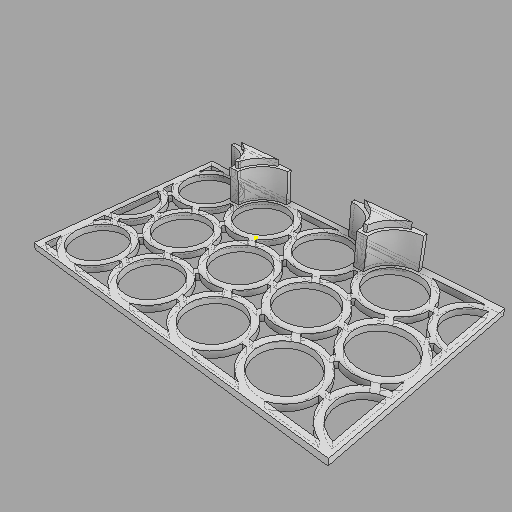
# Autodesk Inventor part: TubeHolder
Saved by Autodesk Inventor 2025 (Build 290162010, 162A)
## iProperties
Created: 2025-03-06
Part Number: TubeHolder
Material: Generic
Document SubType Name: Modeling
Designer: schanen
Density: 1 g/cm^3
Appearance: Default
Author: schanen
Autodesk Inventor part; units mm, degrees
ref_plane "YZ Plane" through (0, 0, 0) normal (1, 0, 0) x (0, 1, 0)
ref_plane "XZ Plane" through (0, 0, 0) normal (0, 1, 0) x (-1, 0, 0)
ref_plane "XY Plane" through (0, 0, 0) normal (0, 0, 1) x (1, 0, 0)
sketch "Sketch1" plane through (0, 0, 0) normal (0, 1, 0) x (-1, 0, 0)
  line L0 (-47.5, 29.5) -> (47.5, 29.5)
  line L1 (47.5, 29.5) -> (47.5, -29.5)
  line L2 (47.5, -29.5) -> (-47.5, -29.5)
  line L3 (-47.5, -29.5) -> (-47.5, 29.5)
  line L4 (-47.5, 29.5) -> (47.5, -29.5) construction
  line L5 (47.5, 29.5) -> (-47.5, -29.5) construction
  circle A0 centre (36.75, -18.1865) radius 8
  line L6 (36.75, -18.1865) -> (23.7803, 4.2776)
  circle A1 centre (26.25, 0) radius 8
  circle A2 centre (15.75, 18.1865) radius 8
  circle A3 centre (15.75, -18.1865) radius 8
  circle A4 centre (5.25, 0) radius 8
  circle A5 centre (-5.25, 18.1865) radius 8
  circle A6 centre (57.75, -18.1865) radius 8
  circle A7 centre (47.25, 0) radius 8
  circle A8 centre (36.75, 18.1865) radius 8
  circle A9 centre (-5.25, -18.1865) radius 8
  circle A10 centre (-15.75, 0) radius 8
  circle A11 centre (-26.25, 18.1865) radius 8
  circle A12 centre (78.75, -18.1865) radius 8
  circle A13 centre (68.25, 0) radius 8
  circle A14 centre (57.75, 18.1865) radius 8
  circle A15 centre (-26.25, -18.1865) radius 8
  circle A16 centre (-36.75, 0) radius 8
  circle A17 centre (-47.25, 18.1865) radius 8
  circle A18 centre (36.75, -18.1865) radius 10
  circle A19 centre (26.25, 0) radius 10
  circle A20 centre (15.75, 18.1865) radius 10
  circle A21 centre (15.75, -18.1865) radius 10
  circle A22 centre (5.25, 0) radius 10
  circle A23 centre (-5.25, 18.1865) radius 10
  circle A24 centre (57.75, -18.1865) radius 10
  circle A25 centre (47.25, 0) radius 10
  circle A26 centre (36.75, 18.1865) radius 10
  circle A27 centre (-5.25, -18.1865) radius 10
  circle A28 centre (-15.75, 0) radius 10
  circle A29 centre (-26.25, 18.1865) radius 10
  circle A30 centre (78.75, -18.1865) radius 10
  circle A31 centre (68.25, 0) radius 10
  circle A32 centre (57.75, 18.1865) radius 10
  circle A33 centre (-26.25, -18.1865) radius 10
  circle A34 centre (-36.75, 0) radius 10
  circle A35 centre (-47.25, 18.1865) radius 10
  line L7 (-45.5, 27.5) -> (45.5, 27.5)
  line L8 (45.5, 27.5) -> (45.5, -27.5)
  line L9 (45.5, -27.5) -> (-45.5, -27.5)
  line L10 (-45.5, -27.5) -> (-45.5, 27.5)
  line L11 (-45.5, 27.5) -> (45.5, -27.5) construction
  line L12 (45.5, 27.5) -> (-45.5, -27.5) construction
  circle A36 centre (99.75, -18.1865) radius 8
  circle A37 centre (89.25, 0) radius 8
  circle A38 centre (78.75, 18.1865) radius 8
  circle A39 centre (-47.25, -18.1865) radius 8
  circle A40 centre (-57.75, 0) radius 8
  circle A41 centre (-68.25, 18.1865) radius 8
  circle A42 centre (99.75, -18.1865) radius 10
  circle A43 centre (89.25, 0) radius 10
  circle A44 centre (78.75, 18.1865) radius 10
  circle A45 centre (-47.25, -18.1865) radius 10
  circle A46 centre (-57.75, 0) radius 10
  circle A47 centre (-68.25, 18.1865) radius 10
  point P0 (0, 0)
  point P1 (45.5, -23.0278)
  point P2 (40.3913, -27.5)
  point P3 (40.3913, 27.5)
  point P4 (45.5, 23.0278)
  point P5 (45.5, -13.3453)
  point P6 (33.1087, -27.5)
  point P7 (19.3913, -27.5)
  point P8 (12.1087, -27.5)
  point P9 (-1.6087, -27.5)
  point P10 (-8.8913, -27.5)
  point P11 (-22.6087, -27.5)
  point P12 (-29.8913, -27.5)
  point P13 (-45.5, -4.8412)
  point P14 (-45.5, 4.8412)
  point P15 (-29.8913, 27.5)
  point P16 (-22.6087, 27.5)
  point P17 (-8.8913, 27.5)
  point P18 (-1.6087, 27.5)
  point P19 (12.1087, 27.5)
  point P20 (19.3913, 27.5)
  point P21 (33.1087, 27.5)
  point P22 (45.5, 13.3453)
  point P23 (-45.5, 25.9928)
  point P24 (-45.5, 10.3803)
  point P25 (-45.5, 8.3408)
  point P26 (-43.6087, 27.5)
  point P27 (-45.5, -8.3408)
  point P28 (-45.5, -10.3803)
  point P29 (-45.5, -25.9928)
  point P30 (-43.6087, -27.5)
  point P31 (45.5, -9.8457)
  point P32 (45.5, -7.8062)
  point P33 (45.5, 7.8062)
  point P34 (45.5, 9.8457)
  dimension "d0" = 95
  dimension "d1" = 59
  dimension "d2" = 16
  dimension "d3" = 60
  dimension "d6" = 21
  dimension "d9" = 21
  dimension "d12" = 11.3135
  dimension "d13" = 10.75
  dimension "d14" = 36.3731
  dimension "d15" = 20
  dimension "d18" = 21
  dimension "d21" = 21
  dimension "d24" = 2
  dimension "d25" = 2
  constraints: 48 centre point, 26 end point, 4 horizontal, 4 midpoint, 4 parallel, 2 perpendicular, 1 coincident, 94 other
  measures "d0" distance of L1.end L2.end
  measures "d1" distance of L0.end L1.end
  measures "d2" diameter of A0
  measures "d3" angle of L2 L6
  measures "d6" distance of L6.start A1.centre
  measures "d9" distance of L6.start A3.centre
  measures "d12" distance from line of L2 L6.start
  measures "d13" distance from line of L1 L6.start
  measures "d14" distance of A11.centre A15.centre
  measures "d15" diameter of A18
  measures "d18" distance of A18.centre A19.centre
  measures "d21" distance of A18.centre A21.centre
  measures "d24" distance between parallel lines of L2 L9
  measures "d25" distance between parallel lines of L1 L8
extrude "Extrusion1" add sketch "Sketch1" along normal blind 2 contours L0 L1 A25 L8 A26 L7 A20 A23 A29 A35 L3 | A35 L7 L10 A17 L3 | L1 A7 L8 A25 | A17 L10 L3 | A35 L10 A17 L7 | A35 L10 A34 A45 L3 | L3 A17 L10 A35 | L1 A7 L8 | L8 A7 A25 | L7 A29 | A29 L7 | A45 L10 A39 L3 | L1 A25 L8 A7 | L1 L2 L3 A45 L9 A33 A27 A21 A18 L8 A25 | L8 A26 | A26 L7 L8 | A39 L10 L3 | A45 L9 L10 A39 | L3 A39 L10 L9 A45 | L10 A34 | A34 L10 | L8 A18 L9 | A18 L8 | A26 L7 | L7 A23 | A23 L7 | L7 A20 | A20 L7 | L9 A33 | A33 L9 | L9 A18 | L9 A21 | A21 L9 | L9 A27 | A27 L9 | A19 | A22 | A28 picked at (36.4286, 27.0427) picked at (36.9961, -27.0508)
sketch "Sketch3" plane through (0, 2, 0) normal (0, 1, 0) x (1, 0, 0)
  circle A0 centre (-36.75, 18.1865) radius 8 projected
  circle A1 centre (-26.25, 0) radius 8 projected
  line L0 (-36.75, 18.1865) -> (-26.25, 0)
  circle A2 centre (-15.75, 18.1865) radius 8 projected
  line L1 (-36.75, 18.1865) -> (-15.75, 18.1865)
  line L2 (-33.6474, 10.8127) -> (-31.0847, 6.3739)
  line L3 (-31.9153, 11.8127) -> (-29.3526, 7.3739)
  arc A3 (-33.6474, 10.8127) -> (-31.9153, 11.8127) centre (-36.75, 18.1865) ccw
  arc A4 (-29.3526, 7.3739) -> (-31.0847, 6.3739) centre (-26.25, 0) ccw
  point P0 (0, 0)
  dimension "d28" = 1
  dimension "d29" = 1
  constraints: 8 end point, 8 point on circle, 2 centre point, 2 coincident, 2 parallel, 1 horizontal
  measures "d28" distance between parallel lines of L0 L2
  measures "d29" distance between parallel lines of L3 L0
extrude "Extrusion2" add sketch "Sketch3" against normal up to surface (2 mm away) contours A0 L0 A1 L2 | L3 A1 L0 A0
pattern_linear "Rectangular Pattern1" count 2 spacing 21 along (0.5, 0, 0.8660254) count 4 spacing 21 along (1, 0, 0) of "Extrusion2"
mirror "Mirror1" about plane through (0, 0, 0) normal (0, 0, 1) of "Extrusion2", "Rectangular Pattern1"
sketch "Sketch5" plane through (0, 2, 0) normal (0, 1, 0) x (1, 0, 0)
  line L0 (-28.8127, 19.1865) -> (-23.6873, 19.1865)
  circle A0 centre (-15.75, 18.1865) radius 8 projected
  circle A1 centre (-36.75, 18.1865) radius 8 projected
  line L1 (-28.8127, 17.1865) -> (-23.6873, 17.1865)
  arc A2 (-28.8127, 17.1865) -> (-28.8127, 19.1865) centre (-36.75, 18.1865) ccw
  arc A3 (-23.6873, 19.1865) -> (-23.6873, 17.1865) centre (-15.75, 18.1865) ccw
  point P0 (0, 0)
  dimension "d38" = 1
  dimension "d39" = 1
  constraints: 8 point on circle, 4 end point, 2 centre point, 2 coincident, 2 horizontal
  measures "d38" distance from line of A1.centre L1
  measures "d39" distance from line of A1.centre L0
extrude "Extrusion3" add sketch "Sketch5" against normal up to surface (2 mm away) contours L0 A0 L1 A1
pattern_linear "Rectangular Pattern2" count 2 spacing 36.3731 along (0, 0, 1) count 4 spacing 21 along (1, 0, 0) of "Extrusion3"
sketch "Sketch6" plane through (0, 2, 0) normal (0, 1, 0) x (1, 0, 0)
  circle A0 centre (36.75, 0) radius 8 projected
  line L0 (28.8127, 1) -> (23.6873, 1)
  circle A1 centre (15.75, 0) radius 8 projected
  line L1 (28.8127, -1) -> (23.6873, -1)
  circle A2 centre (15.75, 0) radius 8 projected
  arc A3 (28.8127, 1) -> (28.8127, -1) centre (36.75, 0) ccw
  arc A4 (23.6873, -1) -> (23.6873, 1) centre (15.75, 0) ccw
  point P0 (0, 0)
  dimension "d48" = 1
  dimension "d49" = 1
  constraints: 8 point on circle, 4 end point, 2 centre point, 2 coincident, 2 horizontal, 1 point on line, 2 other
  measures "d48" distance from line of A0.centre L1
  measures "d49" distance from line of A0.centre L0
extrude "Extrusion4" add sketch "Sketch6" against normal up to surface (2 mm away) contours A0 L1 A1 L0
pattern_linear "Rectangular Pattern3" count 4 spacing 21 along (-1, 0, 0) of "Extrusion4"
sketch "Sketch7" plane through (0, 2, 0) normal (0, 1, 0) x (1, 0, 0)
  circle A0 centre (-36.75, 18.1865) radius 8 projected
  circle A1 centre (-36.75, -18.1865) radius 8 projected
  line L0 (-36.75, 18.1865) -> (-36.75, -18.1865) construction
  line L1 (-32.6411, 9.0697) -> (-32.091, 8.1168) projected
  line L2 (-30.3589, 9.1168) -> (-30.909, 10.0697) projected
  line L3 (-32.6411, -9.0697) -> (-32.091, -8.1168) projected
  line L4 (-30.3589, -9.1168) -> (-30.909, -10.0697) projected
  line L5 (-40.8589, 9.0697) -> (-41.409, 8.1168)
  line L6 (-43.1411, 9.1168) -> (-42.591, 10.0697)
  line L7 (-40.8589, -9.0697) -> (-41.409, -8.1168)
  line L8 (-43.1411, -9.1168) -> (-42.591, -10.0697)
  arc A2 (-45.5, -7.8062) -> (-45.5, 7.8062) centre (-47.25, 0) ccw projected
  arc A3 (-41.409, 8.1168) -> (-43.1411, 9.1168) centre (-47.25, 0) ccw
  arc A4 (-42.591, 10.0697) -> (-40.8589, 9.0697) centre (-36.75, 18.1865) ccw
  arc A5 (-40.8589, -9.0697) -> (-42.591, -10.0697) centre (-36.75, -18.1865) ccw
  arc A6 (-43.1411, -9.1168) -> (-41.409, -8.1168) centre (-47.25, 0) ccw
  point P0 (0, 0)
  constraints: 10 end point, 8 point on circle, 8 symmetric about line, 4 centre point, 4 coincident, 1 vertical
extrude "Extrusion5" add sketch "Sketch7" against normal up to surface (2 mm away) contours L5 A3 L6 A4 | A5 L8 A6 L7
sketch "Sketch8" plane through (0, 2, 0) normal (0, 1, 0) x (1, 0, 0)
  circle A0 centre (-36.75, 18.1865) radius 8 projected
  circle A1 centre (-15.75, 18.1865) radius 8 projected
  line L0 (-36.75, 18.1865) -> (-15.75, 18.1865)
  line L1 (-36.75, 18.1865) -> (-36.75, 28.5)
  line L2 (47.5, 29.5) -> (-47.5, 29.5) projected
  line L3 (-15.75, 18.1865) -> (-15.75, 28.5)
  circle A2 centre (-36.75, 18.1865) radius 9
  circle A3 centre (-15.75, 18.1865) radius 9
  line L4 (-36.75, 28.5) -> (-15.75, 28.5)
  line L5 (-33.1087, 27.5) -> (-19.3913, 27.5) projected
  arc A4 (-26.8001, 19.1865) -> (-33.1087, 27.5) centre (-36.75, 18.1865) ccw projected
  line L6 (-25.6999, 19.1865) -> (-26.8001, 19.1865) projected
  arc A5 (-19.3913, 27.5) -> (-25.6999, 19.1865) centre (-15.75, 18.1865) ccw projected
  point P0 (0, 0)
  point P1 (-36.75, 27.1865)
  point P2 (-27.75, 18.1865)
  point P3 (-24.75, 18.1865)
  point P4 (-15.75, 27.1865)
  dimension "d57" = 1
  dimension "d58" = 18
  dimension "d59" = 18
  constraints: 8 end point, 2 centre point, 2 coincident, 2 horizontal, 2 vertical
  measures "d57" distance from line of L2 L1.end
  measures "d58" diameter of A2
  measures "d59" diameter of A3
extrude "Extrusion6" add sketch "Sketch8" along normal blind 10 contours A2 L1 L4 L3 A3 L0 | L5 A5 L6 A4
pattern_linear "Rectangular Pattern4" count 2 spacing 42 along (1, 0, 0) of "Extrusion6"
sketch "Sketch12" plane through (5.25, 12, -28.5) normal (0, 1, 0) x (1, 0, 0)
  point P0 (-5.25, -28.5)
sketch "Sketch13" plane through (5.25, 12, -28.5) normal (0, 1, 0) x (1, 0, 0)
  arc A0 (9.9499, -9.3135) -> (3.6413, -1) centre (0, -10.3135) ccw projected
  arc A1 (17.3587, -1) -> (11.0501, -9.3135) centre (21, -10.3135) ccw projected
  line L0 (3.6413, -1) -> (17.3587, -1) projected
  arc A2 (-24.6413, -1) -> (-30.9499, -9.3135) centre (-21, -10.3135) ccw projected
  arc A3 (-32.0501, -9.3135) -> (-38.3587, -1) centre (-42, -10.3135) ccw projected
  line L1 (-21, 0) -> (-42, 0) construction
  line L2 (-38.3587, -1) -> (-24.6413, -1) projected
  line L3 (11.0501, -9.3135) -> (9.9499, -9.3135) projected
  line L4 (-30.9499, -9.3135) -> (-32.0501, -9.3135) projected
  point P0 (-5.25, -28.5)
extrude "Extrusion9" add sketch "Sketch13" along normal blind 2
equation "\"d12\" = -0.5 * d14 + 0.5 * d1"
equation "\"d18\" = d6"
equation "\"d21\" = d9"
equation "\"d29\" = d28"
equation "\"d44\" = d14"
equation "\"d59\" = d58"
body "Solid1"
